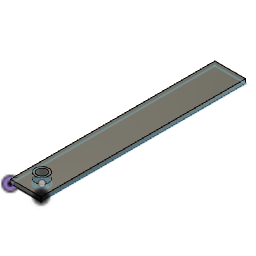
Lid v4 (Autodesk Fusion 360 design; units mm, degrees)
Autodesk Fusion 360 part; units mm, degrees
sketch "Sketch1" plane through (0, 0, 0) normal (0, 1, 0) x (1, 0, 0)
  line L0 (0, 0) -> (38, 0)
  line L1 (38, 0) -> (38, 252.95)
  line L2 (38, 252.95) -> (0, 252.95)
  line L3 (0, 252.95) -> (0, 0)
  line L4 (38, 0, 0) -> (38, 0, 5)
  circle A0 centre (19, 20) radius 6
  circle A1 centre (19, 20) radius 8.5
  dimension "d1" = 38
  dimension "d2" = 252.95
  dimension "d3" = 38
  dimension "d4" = 252.95
  dimension "d5" = 5
  dimension "d9" = 12
  dimension "d10" = 17
  dimension "d21" = 20
  constraint coincident L0.start L3.end
  constraint horizontal L0
  constraint perpendicular L0 L1
  constraint perpendicular L1 L2
  constraint perpendicular L0 L3
  constraint concentric A0 A1
  measures "d1" distance of L0.start L0.end
  measures "d2" distance of L0.end L1.end
  measures "d3" distance of L1.end L2.end
  measures "d4" distance of L2.end L0.start
  measures "d5" distance of L0.end L1.start
  measures "d9" diameter of A0
  measures "d10" diameter of A1
  measures "d21" distance of L0 A0.centre
extrude "Extrude1" add sketch "Sketch1" along normal blind 5 contours L0 L1 L2 L3 | A0 | A1 makes body 1
extrude "Extrude2" cut 1 faces at (12.6667, 5, -168.6333) along direction (0, -1, 0) blind 5000 on bodies 1 bodies 1
extrude "Extrude3" add sketch "Sketch1" along normal blind 8 contours A1 bodies 1
extrude "Extrude4" add sketch "Sketch1" along normal blind 5 contours L0 L1 L2 L3 bodies 1
extrude "Extrude5" add 1 faces at (26.6127, 8, -19.2796) along direction (0, 1, 0) blind 2 on bodies 1 bodies 1
extrude "Extrude6" add 1 faces at (26.6127, 10, -19.2796) along direction (0, 1, 0) blind 2 on bodies 1 bodies 1
copy_body "Body->Comp1" bodies 1 removing the originals makes body 2 in component "Lid"
component "Lid" placed x (1, 0, 0) y (0, 1, 0) z (0, 0, 1) at (0, 0, 0)
